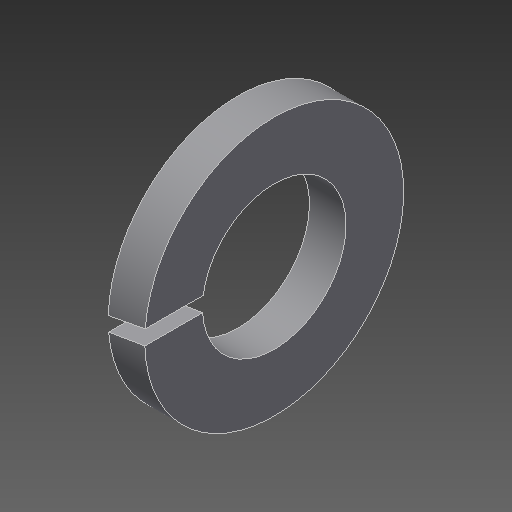
# Autodesk Inventor part: SLW5
Saved by Autodesk Inventor 2021.1 (Build 251245010, 245A)
## iProperties
Created: 2010-03-07
Part Number: SLW5
Catalog Web Link: www.cadenas.de
Document SubType Name: Modeling
Density: 1 g/cm^3
Material: MISUMI
Appearance: 既定
Category: PARTsolutions
NB: SLW5
NN: SLW, SSLW
NT: Spring Washers
NBSYN: $PN.
LINA: SLW5
PN: SLW5
ST: Trivalent Chromate Plating
NO: 5
DD: 5.1
D: 9.2
TT: 1.3
M1: 5.000
KT: DUMMY
PSOL_IDENT_0: {\\10.0.0.149\dplatte\cadenas\23d-libs\misumi\metric\27_screws_nuts\slw.prj},156 {VTYP=3D},{NB=SLW5}
PSOL_IDENT_1: ,{LINA=SLW5},{NN=SLW, SSLW},{DATE=26.08.2009 09:13:32},{GEOMDATE=07.07.2009 12:27:00},{VERSION=},{LI
PSOL_IDENT_2: NEID=40},{LINESUBID=-1},{WBVAR=MAT}  {NB=SLW5},{LINA=SLW5},{KT=DUMMY},{PN=SLW5},{MAT=},{ST=Trivalent
PSOL_IDENT_3: Chromate Plating},{NO=5},{DD=5.1},{D=9.2},{TT=1.3},{M1=5.000}
Title: ばね座金
Comments: Spring Washers
Autodesk Inventor part; units mm, degrees
sketch "Sketch_1" plane through (0, 0, 0) normal (0, 0, 1) x (1, 0, 0)
  line L0 (0.65, 0) -> (-0.65, 0)
  line L1 (-0.65, 2.55) -> (0.65, 2.55)
  line L2 (0.65, 2.55) -> (0.65, 4.6)
  line L3 (0.65, 4.6) -> (-0.65, 4.6)
  line L4 (-0.65, 4.6) -> (-0.65, 2.55)
  constraints: 10 end point
revolve "Revolution1" add sketch "Sketch_1" angle 360 about axis through (0.65, 0, 0) along (-1, 0, 0)
sketch "Sketch_2" plane through (0, 0, 0) normal (0, 0, 1) x (1, 0, 0)
  line L0 (-1.3245, 0.0254) -> (-1.236, -0.4769)
  line L1 (-1.236, -0.4769) -> (1.3245, -0.0254)
  line L2 (1.3245, -0.0254) -> (1.236, 0.4769)
  line L3 (1.236, 0.4769) -> (-1.3245, 0.0254)
  constraints: 8 end point
extrude "Extrusion1" cut sketch "Sketch_2" along normal blind 9.2
ref_plane "spring_washer_to_bolt_XY" through (0, 0, 0) normal (1, 0, 0) x (0, 0, -1)
ref_plane "spring_washer_to_bolt_YZ" through (0, 0, 0) normal (0, 0, -1) x (0, 1, 0)
ref_plane "spring_washer_to_bolt_ZX" through (0, 0, 0) normal (0, 1, 0) x (1, 0, 0)
